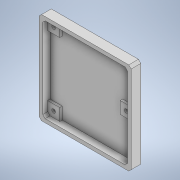
# Autodesk Inventor part: aluminium_block
Saved by Autodesk Inventor 2020.3 (Build 243373000, 373)
## iProperties
Created: 2020-07-08
Part Number: aluminium_block
Material: Generic
Document SubType Name: Modeling
Designer: OskarJohansson
Density: 1 g/cm^3
Appearance: Default
Author: OskarJohansson
Autodesk Inventor part; units mm, degrees
ref_plane "YZ Plane" through (0, 0, 0) normal (1, 0, 0) x (0, 1, 0)
ref_plane "XZ Plane" through (0, 0, 0) normal (0, 1, 0) x (-1, 0, 0)
ref_plane "XY Plane" through (0, 0, 0) normal (0, 0, 1) x (1, 0, 0)
sketch "Sketch1" plane through (0, 0, 0) normal (0, 0, 1) x (1, 0, 0)
  line L0 (-38, -38) -> (38, -38)
  line L1 (38, -38) -> (38, 38)
  line L2 (38, 38) -> (-38, 38)
  line L3 (-38, 38) -> (-38, -38)
  line L4 (-38, -38) -> (38, 38) construction
  line L5 (38, -38) -> (-38, 38) construction
  line L6 (-30, 35) -> (30, 35) projected
  line L7 (-35, -30) -> (-35, 30) projected
  line L8 (35, 30) -> (35, -30) projected
  line L9 (30, -35) -> (-30, -35) projected
  point P0 (0, 0)
  dimension "d0" = 3
  dimension "d1" = 3
  constraints: 12 end point, 2 midpoint, 2 parallel, 1 horizontal, 1 perpendicular
  measures "d0" distance between parallel lines of L2 L6
  measures "d1" distance between parallel lines of L1 L8
extrude "Extrusion1" add sketch "Sketch1" along normal blind 3 and the other way blind 5
sketch "Sketch2" plane through (0, 0, 3) normal (0, 0, 1) x (1, 0, 0)
  line L0 (35, -35) -> (-35, -35)
  line L1 (-35, -35) -> (-35, 35)
  line L2 (-35, 35) -> (35, 35)
  line L3 (35, 35) -> (35, -35)
  line L4 (35, -35) -> (-35, 35) construction
  line L5 (-35, -35) -> (35, 35) construction
  point P0 (0, 0)
  dimension "d6" = 70
  dimension "d7" = 70
  constraints: 12 end point, 2 midpoint, 2 parallel, 1 horizontal, 1 perpendicular
  measures "d6" distance of L0.end L1.end
  measures "d7" distance of L1.end L2.end
extrude "Extrusion2" cut sketch "Sketch2" against normal blind 6
sketch "Sketch3" plane through (0, 0, -3) normal (0, 0, 1) x (1, 0, 0)
  line L0 (-25, 25) -> (-35, 25)
  line L1 (-35, 25) -> (-35, 35)
  line L2 (-35, 35) -> (-25, 35)
  line L3 (-25, 35) -> (-25, 25)
  line L4 (-25, 25) -> (-35, 35) construction
  line L5 (-35, 25) -> (-25, 35) construction
  line L6 (-35, -35) -> (-35, 35) projected
  line L7 (-35, 35) -> (35, 35) projected
  point P0 (0, 0)
  point P1 (-30, 30)
  dimension "d10" = 10
  dimension "d11" = 10
  constraints: 12 end point, 2 collinear, 2 midpoint, 2 parallel, 1 horizontal, 1 perpendicular
  measures "d10" distance of L0.start L0.end
  measures "d11" distance of L2.end L0.start
extrude "Extrusion3" add sketch "Sketch3" along normal blind 2
sketch "Sketch4" plane through (0, 0, -3) normal (0, 0, 1) x (1, 0, 0)
  line L0 (25, -5) -> (35, -5)
  line L1 (35, -5) -> (35, 5)
  line L2 (35, 5) -> (25, 5)
  line L3 (25, 5) -> (25, -5)
  line L4 (25, -5) -> (35, 5) construction
  line L5 (35, -5) -> (25, 5) construction
  line L6 (-53.2, 0) -> (53.2, 0) projected
  line L7 (35, 35) -> (35, -35) projected
  point P0 (0, 0)
  point P1 (30, 0)
  point P2 (30, 0)
  dimension "d23" = 10
  dimension "d24" = 10
  constraints: 12 end point, 3 midpoint, 2 parallel, 1 collinear, 1 horizontal, 1 perpendicular, 1 point on line
  measures "d23" distance of L1.end L2.end
  measures "d24" distance of L0.end L1.end
extrude "Extrusion4" add sketch "Sketch4" along normal up to surface (2 mm away)
hole "Hole1" at (-30, 30, -1) direction (0, 0, -1) diameter 3 end through all
mirror "Mirror1" about plane through (0, 0, 0) normal (0, 1, 0) of "Extrusion3", "Hole1"
hole "Hole2" at (30, 0, -1) direction (0, 0, -1) diameter 3 end through all
chamfer "Chamfer1" distance 2 angle 45 8 edges at (38, 38, -1) (35, 35, 0) (38, -38, -1) (35, -35, 0) (-35, -35, 1) (-38, -38, -1) (-38, 38, -1) (-35, 35, 1)
equation "\"d1\" = d0"
equation "\"d7\" = d6"
equation "\"d24\" = d23"
body "Solid1"
